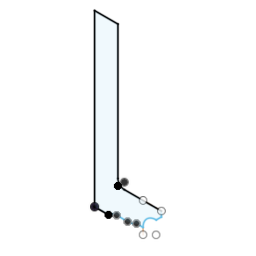
Muototerä3 (Autodesk Fusion 360 design; units mm, degrees)
Autodesk Fusion 360 part; units mm, degrees
sketch "Sketch1" plane through (0, 0, 0) normal (0, 0, 1) x (1, 0, 0)
  line L0 (0, 0) -> (0, 46.3)
  line L1 (0, 46.3) -> (6.35, 46.3)
  line L2 (6.35, 46.3) -> (6.35, 9.85)
  line L3 (8.1, 8.1) -> (18.2, 8.1)
  arc A0 (6.35, 9.85) -> (8.1, 8.1) centre (8.1, 9.85) ccw
  line L4 (18.2, 8.1) -> (18.2, 6.7)
  line L5 (18.2, 6.7) -> (16.8, 5.3)
  line L6 (13.2, 0) -> (13.2, 1.75) construction
  line L7 (13.2, 8.1) -> (18.2, 8.1) construction
  arc A1 (16.8, 5.3) -> (13.2, 1.75) centre (16.7503, 1.75) ccw
  line L8 (0, 0) -> (3.8, 0) construction
  line L9 (13.2, 1.75) -> (11.4, 1.75)
  spline S0 degree 5 poles (3.8, 0) (3.874, 0.0724) (4.0254, 0.2108) (4.2632, 0.3991) (4.6016, 0.6114) (5.0606, 0.8115) (5.5553, 0.947) (6.0834, 1.0219) (6.6399, 1.0454) (7.2162, 1.0336) (7.8014, 1.0063) (8.3841, 0.9843) (8.9535, 0.9874) (9.5011, 1.0314) (10.0218, 1.1255) (10.5134, 1.274) (10.8827, 1.437) (11.1465, 1.584) (11.3165, 1.6928) (11.4, 1.75) knots 0 0 0 0 0 0 0.066667 0.133333 0.2 0.266667 0.333333 0.4 0.466667 0.533333 0.6 0.666667 0.733333 0.8 0.866667 0.933333 1 1 1 1 1 1
  line L10 (6, 1) -> (5.4739, 0.9123)
  line L11 (0, 0) -> (3.8, 0)
  point P0 (6.35, 8.1)
  point P1 (9, 1)
  dimension "d1" = 46.3
  dimension "d2" = 6.35
  dimension "d3" = 38.2
  dimension "d11" = 1.75
  dimension "d12" = 1.4
  dimension "d16" = 6.35
  dimension "d17" = 3.8
  dimension "d18" = 1.8
  constraint coincident L0.start L8.start
  constraint vertical L0
  constraint perpendicular L0 L1
  constraint perpendicular L1 L2
  constraint perpendicular L0 L11
  constraint perpendicular L2 L3
  constraint coincident P0 L2
  constraint coincident P0 L3
  constraint tangent L2 A0
  constraint tangent L3 A0
  constraint perpendicular L3 L4
  constraint vertical L6
  constraint horizontal L7
  constraint tangent L6 A1
  constraint perpendicular L0 L8
  constraint perpendicular L6 L9
  constraint coincident S0 L10.end
  measures "d1" distance of L0.start L0.end
  measures "d2" distance of L0.end L1.end
  measures "d3" distance of L1.end P0
  measures "d11" radius of A0
  measures "d12" distance of L3.end L4.end
  measures "d16" distance of L7.start L6.end
  measures "d17" distance of L0.start L8.end
  measures "d18" distance of L6.end L9.end
revolve "Revolve1" add sketch "Sketch1" angle 360 about axis through (0, 0, 0) along (0, 1, 0) contours L0 L1 L2 L3 A0 L4 L5 A1 L9 S0 L11
